Autodesk Inventor part; units mm, degrees
(part 2 of 2)
  spline S94 degree 2 poles (-16.0777, 89.9073) (-16.1789, 89.9073) (-16.3568, 89.927) (-16.4235, 89.9493) knots 0 0 0 1 2 2 2
  line L146 (-16.4235, 89.9493) -> (-16.4235, 90.342)
  line L147 (-16.4235, 90.342) -> (-16.4062, 90.342)
  spline S95 degree 2 poles (-16.4062, 90.342) (-16.3494, 90.3124) (-16.1419, 90.2605) (-16.0233, 90.2605) knots 0 0 0 1 2 2 2
  spline S96 degree 2 poles (-16.0233, 90.2605) (-15.643, 90.2605) (-15.1761, 90.7743) (-15.1317, 91.2781) knots 0 0 0 1 2 2 2
  spline S97 degree 2 poles (-15.1317, 91.2781) (-15.2774, 91.1769) (-15.5837, 91.0657) (-15.7665, 91.0657) knots 0 0 0 1 2 2 2
  spline S98 degree 2 poles (-15.7665, 91.0657) (-15.9443, 91.0657) (-16.2111, 91.1374) (-16.3568, 91.246) knots 0 0 0 1 2 2 2
  spline S99 degree 2 poles (-16.3568, 91.246) (-16.5248, 91.372) (-16.6878, 91.7623) (-16.6878, 92.0241) knots 0 0 0 1 2 2 2
  spline S100 degree 2 poles (-16.2728, 92.0414) (-16.2728, 91.8537) (-16.174, 91.5992) (-16.0653, 91.5103) knots 0 0 0 1 2 2 2
  spline S101 degree 2 poles (-16.0653, 91.5103) (-15.9838, 91.4461) (-15.7813, 91.4041) (-15.6751, 91.4041) knots 0 0 0 1 2 2 2
  spline S102 degree 2 poles (-15.6751, 91.4041) (-15.5318, 91.4041) (-15.2626, 91.4906) (-15.1317, 91.5721) knots 0 0 0 1 2 2 2
  spline S103 degree 2 poles (-15.1317, 91.5721) (-15.1292, 91.6165) (-15.1243, 91.7005) (-15.1243, 91.7647) knots 0 0 0 1 2 2 2
  spline S104 degree 2 poles (-15.1243, 91.7647) (-15.1243, 92.0809) (-15.2478, 92.4687) (-15.3416, 92.57) knots 0 0 0 1 2 2 2
  spline S105 degree 2 poles (-15.3416, 92.57) (-15.4281, 92.6663) (-15.6158, 92.7429) (-15.722, 92.7429) knots 0 0 0 1 2 2 2
  spline S106 degree 2 poles (-15.722, 92.7429) (-15.969, 92.7429) (-16.2728, 92.3921) (-16.2728, 92.0414) knots 0 0 0 1 2 2 2
  line L148 (-17.7029, 93.0121) -> (-17.2139, 93.0121)
  line L149 (-17.2139, 93.0121) -> (-17.2139, 92.4292)
  line L150 (-17.2139, 92.4292) -> (-17.7029, 92.4292)
  line L151 (-17.7029, 92.4292) -> (-17.7029, 93.0121)
  line L152 (-20.1977, 93.0121) -> (-18.318, 93.0121)
  line L153 (-18.318, 93.0121) -> (-18.318, 92.5798)
  spline S107 degree 2 poles (-18.318, 92.5798) (-18.5205, 92.3897) (-18.8811, 92.0364) (-19.054, 91.8463) knots 0 0 0 1 2 2 2
  spline S108 degree 2 poles (-19.054, 91.8463) (-19.4023, 91.4634) (-19.6567, 91.004) (-19.6567, 90.7594) knots 0 0 0 1 2 2 2
  spline S109 degree 2 poles (-19.6567, 90.7594) (-19.6567, 90.631) (-19.5777, 90.4383) (-19.5061, 90.3766) knots 0 0 0 1 2 2 2
  spline S110 degree 2 poles (-19.5061, 90.3766) (-19.4344, 90.3148) (-19.2467, 90.2531) (-19.1331, 90.2531) knots 0 0 0 1 2 2 2
  spline S111 degree 2 poles (-19.1331, 90.2531) (-19.0244, 90.2531) (-18.8021, 90.3074) (-18.7008, 90.3494) knots 0 0 0 1 2 2 2
  spline S112 degree 2 poles (-18.7008, 90.3494) (-18.6144, 90.384) (-18.4538, 90.4828) (-18.4044, 90.5174) knots 0 0 0 1 2 2 2
  line L154 (-18.4044, 90.5174) -> (-18.3822, 90.5174)
  line L155 (-18.3822, 90.5174) -> (-18.3822, 90.0827)
  spline S113 degree 2 poles (-18.3822, 90.0827) (-18.5082, 90.0209) (-18.9602, 89.8999) (-19.1627, 89.8999) knots 0 0 0 1 2 2 2
  spline S114 degree 2 poles (-19.1627, 89.8999) (-19.59, 89.8999) (-20.0717, 90.3519) (-20.0717, 90.7372) knots 0 0 0 1 2 2 2
  spline S115 degree 2 poles (-20.0717, 90.7372) (-20.0717, 90.9175) (-19.9877, 91.2189) (-19.9136, 91.3473) knots 0 0 0 1 2 2 2
  spline S116 degree 2 poles (-19.9136, 91.3473) (-19.8395, 91.4807) (-19.6246, 91.7425) (-19.5061, 91.8685) knots 0 0 0 1 2 2 2
  spline S117 degree 2 poles (-19.5061, 91.8685) (-19.3134, 92.0784) (-18.8416, 92.528) (-18.7008, 92.6589) knots 0 0 0 1 2 2 2
  line L156 (-18.7008, 92.6589) -> (-20.1977, 92.6589)
  line L157 (-20.1977, 92.6589) -> (-20.1977, 93.0121)
  spline S118 degree 2 poles (-22.4528, 92.0439) (-22.4528, 92.2637) (-22.312, 92.6391) (-22.1836, 92.7774) knots 0 0 0 1 2 2 2
  spline S119 degree 2 poles (-22.1836, 92.7774) (-22.0551, 92.9158) (-21.6723, 93.0763) (-21.4351, 93.0763) knots 0 0 0 1 2 2 2
  spline S120 degree 2 poles (-21.4351, 93.0763) (-21.2178, 93.0763) (-20.7929, 92.98) (-20.6373, 92.9034) knots 0 0 0 1 2 2 2
  line L158 (-20.6373, 92.9034) -> (-20.6373, 92.4712)
  line L159 (-20.6373, 92.4712) -> (-20.667, 92.4712)
  spline S121 degree 2 poles (-20.667, 92.4712) (-20.7139, 92.5057) (-20.8893, 92.5947) (-20.9955, 92.6342) knots 0 0 0 1 2 2 2
  spline S122 degree 2 poles (-20.9955, 92.6342) (-21.1165, 92.6762) (-21.3166, 92.7231) (-21.4426, 92.7231) knots 0 0 0 1 2 2 2
  spline S123 degree 2 poles (-21.4426, 92.7231) (-21.5661, 92.7231) (-21.7982, 92.6342) (-21.8822, 92.5379) knots 0 0 0 1 2 2 2
  spline S124 degree 2 poles (-21.8822, 92.5379) (-21.9588, 92.4465) (-22.0378, 92.2044) (-22.0378, 92.0414) knots 0 0 0 1 2 2 2
  spline S125 degree 2 poles (-22.0378, 92.0414) (-22.0378, 91.8784) (-21.9489, 91.6709) (-21.8649, 91.6017) knots 0 0 0 1 2 2 2
  spline S126 degree 2 poles (-21.8649, 91.6017) (-21.7785, 91.5251) (-21.5216, 91.4609) (-21.366, 91.4609) knots 0 0 0 1 2 2 2
  spline S127 degree 2 poles (-21.366, 91.4609) (-21.198, 91.4609) (-20.8646, 91.5128) (-20.7633, 91.535) knots 0 0 0 1 2 2 2
  line L160 (-20.7633, 91.535) -> (-20.7633, 89.9641)
  line L161 (-20.7633, 89.9641) -> (-22.4355, 89.9641)
  line L162 (-22.4355, 89.9641) -> (-22.4355, 90.3222)
  line L163 (-22.4355, 90.3222) -> (-21.156, 90.3222)
  line L164 (-21.156, 90.3222) -> (-21.156, 91.1349)
  spline S128 degree 2 poles (-21.156, 91.1349) (-21.2301, 91.125) (-21.3734, 91.1176) (-21.4327, 91.1176) knots 0 0 0 1 2 2 2
  spline S129 degree 2 poles (-21.4327, 91.1176) (-21.6673, 91.1176) (-21.9909, 91.1942) (-22.1391, 91.3078) knots 0 0 0 1 2 2 2
  spline S130 degree 2 poles (-22.1391, 91.3078) (-22.2898, 91.4214) (-22.4528, 91.7672) (-22.4528, 92.0439) knots 0 0 0 1 2 2 2
  point P0 (-47.5, 53.2457)
  constraints: 2 other
extrude "Extrusion47" add sketch "Sketch58" along normal blind 1
sketch "Sketch59" plane through (69.5, 80.5, 0) normal (0, 0, -1) x (-1, 0, 0)
  line L0 (124.232, -148.2248) -> (124.232, -65.5994) projected
  line L1 (124.232, -131.7625) -> (22.225, -131.7625)
  line L2 (22.225, -144.4625) -> (124.232, -144.4625)
  line L3 (124.232, -144.4625) -> (124.232, -131.7625)
  line L4 (22.225, -144.4625) -> (19.05, -144.4625)
  line L5 (19.05, -144.4625) -> (19.05, -131.7625)
  line L6 (19.05, -131.7625) -> (22.225, -131.7625)
  point P0 (69.5, -80.5)
  point P1 (22.225, -131.7625)
  constraints: 12 end point, 2 horizontal, 2 parallel, 1 perpendicular, 1 point on line
extrude "Extrusion48" add sketch "Sketch59" against normal blind 1
extrude "Extrusion49" cut sketch "Sketch57" against normal blind 3 contours A0 | A2 | A4 | A5 | A7 | A9
body "Solid1"
